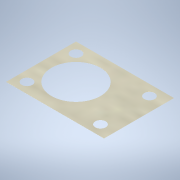
# Autodesk Inventor part: ZYLINDERKOPFDICHTUNG PART 4
Saved by Autodesk Inventor 2022 (Build 260153000, 153)
## iProperties
Created: 2020-07-10
Part Number: ZYLINDERKOPFDICHTUNG PART 4
Material: Paper
Document SubType Name: Modeling
Designer: Smit Ambardekar
Density: 0.93 g/cm^3
Appearance: Cardboard - Chipboard
Author: Smit Ambardekar
Autodesk Inventor part; units mm, degrees
ref_plane "YZ Plane" through (0, 0, 0) normal (1, 0, 0) x (0, 1, 0)
ref_plane "XZ Plane" through (0, 0, 0) normal (0, 1, 0) x (-1, 0, 0)
ref_plane "XY Plane" through (0, 0, 0) normal (0, 0, 1) x (1, 0, 0)
sketch "Sketch1" plane through (0, 0, 0) normal (0, 1, 0) x (-1, 0, 0)
  line L0 (-14, -10) -> (-14, 10)
  line L1 (-14, 10) -> (14, 10)
  line L2 (14, 10) -> (14, -10)
  line L3 (14, -10) -> (-14, -10)
  circle A0 centre (11, -7) radius 1.5
  circle A1 centre (-10, -7) radius 1.5
  circle A2 centre (-10, 7) radius 1.5
  circle A3 centre (11, 7) radius 1.5
  point P0 (0, 0)
  dimension "d0" = 28
  dimension "d1" = 20
  dimension "d6" = 3
  dimension "d7" = 3
  constraints: 8 end point, 4 centre point, 1 horizontal, 1 parallel
  measures "d0" distance of L0.end L1.end
  measures "d1" distance of L0.start L0.end
  measures "d6" diameter of A0
  measures "d7" diameter of A1
extrude "Extrusion1" add sketch "Sketch1" along normal blind 0.01
sketch "Sketch2" plane through (0, 0.01, 0) normal (0, 1, 0) x (1, 0, 0)
  arc A0 (2.7082, 2) -> (2.7082, -2) centre (-4, 0) ccw projected
  circle A1 centre (-4, 0) radius 7
  point P0 (0, 0)
  point P1 (2.7082, -2)
  point P2 (2.7082, 2)
  constraints: 1 centre point, 1 coincident, 1 concentric
extrude "Extrusion2" cut sketch "Sketch2" against normal blind 0.5
body "Solid1"
